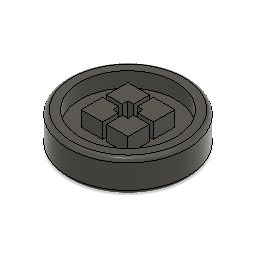
DC801-BM-Joy-Hats-symbols v13 (Autodesk Fusion 360 design; units mm, degrees)
Autodesk Fusion 360 part; units mm, degrees
note: some values were not read from the file. Chosen so that the rebuilt part matches the saved one: which bodies a step acts on; which face or edge a step refers to. Set by a fixed rule: which sketch regions a step uses.
sketch "Sketch1" plane through (0, 0, 0) normal (0, 1, 0) x (1, 0, 0)
  line L0 (0.95, 0.95) -> (-0.95, 0.95)
  line L1 (-0.95, 0.95) -> (-0.95, -0.95)
  line L2 (-0.95, -0.95) -> (0.95, -0.95)
  line L3 (0.95, -0.95) -> (0.95, 0.95)
  line L4 (0.95, 0.95) -> (-0.95, -0.95) construction
  line L5 (-0.95, 0.95) -> (0.95, -0.95) construction
  circle A0 centre (0, 0) radius 7.5
  line L6 (0.25, -2.95) -> (-0.25, -2.95)
  line L7 (-0.25, -2.95) -> (-0.25, 2.95)
  line L8 (-0.25, 2.95) -> (0.25, 2.95)
  line L9 (0.25, 2.95) -> (0.25, -2.95)
  line L10 (0.25, -2.95) -> (-0.25, 2.95) construction
  line L11 (-0.25, -2.95) -> (0.25, 2.95) construction
  line L12 (2.95, 2.95) -> (-2.95, 2.95)
  line L13 (-2.95, 2.95) -> (-2.95, -2.95)
  line L14 (-2.95, -2.95) -> (2.95, -2.95)
  line L15 (2.95, -2.95) -> (2.95, 2.95)
  circle A1 centre (0, 0) radius 6
  line L16 (2.95, 0.25) -> (-2.95, 0.25)
  line L17 (-2.95, 0.25) -> (-2.95, -0.25)
  line L18 (-2.95, -0.25) -> (2.95, -0.25)
  line L19 (2.95, -0.25) -> (2.95, 0.25)
  line L20 (2.95, 0.25) -> (-2.95, -0.25) construction
  line L21 (-2.95, 0.25) -> (2.95, -0.25) construction
  dimension "d1" = 1.9
  dimension "d2" = 1.9
  dimension "d3" = 15
  dimension "d35" = 0.5
  dimension "d63" = 2
  dimension "d68" = 2
  dimension "d71" = 0.5
  dimension "d94" = 5.9
  dimension "d96" = 5.9
  constraint horizontal L0
  constraint perpendicular L0 L1
  constraint parallel L0 L2
  constraint parallel L1 L3
  constraint coincident L4 A0.centre
  constraint coincident L5 A0.centre
  constraint coincident A0.centre A1.centre
  constraint horizontal L6
  constraint perpendicular L6 L7
  constraint parallel L6 L8
  constraint parallel L7 L9
  constraint coincident L10 A0.centre
  constraint coincident L11 A0.centre
  constraint horizontal L16
  constraint perpendicular L16 L17
  constraint parallel L16 L18
  constraint parallel L17 L19
  constraint coincident L20 A0.centre
  constraint coincident L21 A0.centre
  measures "d1" distance of L1.end L2.end
  measures "d2" distance of L0.end L1.end
  measures "d3" diameter of A0
  measures "d35" distance of L7.end L8.end
  measures "d63" distance of L2 L6
  measures "d71" distance of L16.end L17.end
  measures "d94" distance of L16.start L16.end
  measures "d96" distance of L6.start L8.end
extrude "Extrude1" add sketch "Sketch1" along normal blind 3 contours L0 L3 L9 L12 L15 L16 | L0 L1 L7 L12 L13 L16 | L2 L3 L9 L14 L15 L18 | L1 L2 L7 L13 L14 L18 | A0 makes body 1 at (2.95, 1, -1.15) makes body 2 at (2.95, 1, 2.05) makes body 3 at (-1.15, 1, -2.95) makes body 4 at (7.4907, 2, 0.3738) makes body 5 at (-2.95, 1, 1.15)
extrude "Extrude12" add sketch "Sketch1" against normal blind 1 contours L0 L3 L9 L16 | L0 L3 L9 L12 L15 L16 | L0 L7 L9 L16 | L0 L7 L8 L9 L12 | L3 L15 L16 L18 L19 | L3 L9 L16 L18 | L0 L1 L7 L16 | L0 L1 L7 L12 L13 L16 | L7 L9 L16 L18 | L2 L3 L9 L14 L15 L18 | L2 L3 L9 L18 | L1 L7 L16 L18 | L2 L7 L9 L18 | L1 L13 L16 L17 L18 | L1 L2 L7 L18 | L2 L6 L7 L9 L14 | L1 L2 L7 L13 L14 L18 | A0 | A1 bodies 1 2 3 4 5
sketch "Sketch17" plane through (0, 0, 0) normal (0, 1, 0) x (-1, 0, 0)
  line L0 (-2.95, -2.95) -> (-2.95, -0.25)
  line L1 (-2.95, -0.25) -> (-0.95, -0.25)
  line L2 (-0.95, -0.25) -> (-0.95, -0.95)
  line L3 (-0.95, -0.95) -> (-0.25, -0.95)
  line L4 (-0.25, -0.95) -> (-0.25, -2.95)
  line L5 (-0.25, -2.95) -> (-2.95, -2.95)
  line L6 (2.95, -2.95) -> (0.25, -2.95)
  line L7 (0.25, -2.95) -> (0.25, -0.95)
  line L8 (0.25, -0.95) -> (0.95, -0.95)
  line L9 (0.95, -0.95) -> (0.95, -0.25)
  line L10 (0.95, -0.25) -> (2.95, -0.25)
  line L11 (2.95, -0.25) -> (2.95, -2.95)
  line L12 (2.95, 2.95) -> (2.95, 0.25)
  line L13 (2.95, 0.25) -> (0.95, 0.25)
  line L14 (0.95, 0.25) -> (0.95, 0.95)
  line L15 (0.95, 0.95) -> (0.25, 0.95)
  line L16 (0.25, 0.95) -> (0.25, 2.95)
  line L17 (0.25, 2.95) -> (2.95, 2.95)
  line L18 (-2.95, 2.95) -> (-0.25, 2.95)
  line L19 (-0.25, 2.95) -> (-0.25, 0.95)
  line L20 (-0.25, 0.95) -> (-0.95, 0.95)
  line L21 (-0.95, 0.95) -> (-0.95, 0.25)
  line L22 (-0.95, 0.25) -> (-2.95, 0.25)
  line L23 (-2.95, 0.25) -> (-2.95, 2.95)
  line L24 (-2.95, -2.95) -> (2.95, -2.95)
  line L25 (2.95, -2.95) -> (2.95, 2.95)
  line L26 (2.95, 2.95) -> (-2.95, 2.95)
  line L27 (-2.95, 2.95) -> (-2.95, -2.95)
  line L28 (-2.95, -2.95) -> (2.95, 2.95) construction
  line L29 (2.95, -2.95) -> (-2.95, 2.95) construction
  circle A0 centre (0, 0) radius 6
  dimension "d103" = 5.9
  dimension "d104" = 5.9
  constraint horizontal L24
  constraint perpendicular L24 L25
  constraint parallel L24 L26
  constraint parallel L25 L27
  constraint coincident L28 A0.centre
  constraint coincident L29 A0.centre
  measures "d103" distance of L12.start L18.start
  measures "d104" distance of L6.start L12.start
extrude "Extrude18" add sketch "Sketch17" along normal blind 1.1 contours L1 L2 L3 L4 L7 L8 L9 L10 L13 L14 L15 L16 L19 L20 L21 L22 L24 L25 L26 L27 bodies 1
sketch "Sketch18" plane through (0, -1, 0) normal (0, -1, 0) x (1, 0, 0)
  line L0 (6.5, 1.5) -> (-6.5, 1.5)
  line L1 (-6.5, 1.5) -> (-6.5, -1.5)
  line L2 (-6.5, -1.5) -> (6.5, -1.5)
  line L3 (6.5, -1.5) -> (6.5, 1.5)
  line L4 (6.5, 1.5) -> (-6.5, -1.5) construction
  line L5 (-6.5, 1.5) -> (6.5, -1.5) construction
  line L6 (-3.5, 1.5) -> (-3.5, -1.5)
  line L7 (-3.5, 0) -> (-6.5, 0) construction
  line L8 (-3.8606, 0.9565) -> (-6.1403, -0.9573) construction
  line L9 (-6.1151, 1.0426) -> (-4.1467, -0.7978) construction
  circle A0 centre (5, 0) radius 1.5
  line L10 (-0.012, 6.5) -> (-1.7598, 3.5092)
  line L11 (-1.7598, 3.5092) -> (1.7042, 3.4909)
  line L12 (1.7042, 3.4909) -> (-0.012, 6.5)
  circle A1 centre (5, 0) radius 1.1
  line L13 (-4, 1) -> (-6, 1)
  line L14 (-6, 1) -> (-6, -1)
  line L15 (-6, -1) -> (-4, -1)
  line L16 (-4, -1) -> (-4, 1)
  line L17 (-4, 1) -> (-6, -1) construction
  line L18 (-6, 1) -> (-4, -1) construction
  line L19 (-0.0147, 6) -> (-1.3255, 3.7569)
  line L20 (-1.3255, 3.7569) -> (1.2725, 3.7432)
  line L21 (1.2725, 3.7432) -> (-0.0147, 6)
  line L22 (1, -4) -> (-1, -4) construction
  line L23 (-1, -4) -> (-1, -6) construction
  line L24 (-1, -6) -> (1, -6) construction
  line L25 (1, -6) -> (1, -4) construction
  line L26 (1, -4) -> (-1, -6) construction
  line L27 (-1, -4) -> (1, -6) construction
  line L28 (-1, -5.6818) -> (0.6818, -4)
  line L29 (-0.6818, -6) -> (1, -4.3182)
  line L30 (-0.6818, -4) -> (1, -5.6818)
  line L31 (-1, -4.3182) -> (0.6818, -6)
  line L32 (1.5, -3.5) -> (-1.5, -3.5)
  line L33 (-1.5, -3.5) -> (-1.5, -6.5)
  line L34 (-1.5, -6.5) -> (1.5, -6.5)
  line L35 (1.5, -6.5) -> (1.5, -3.5)
  line L36 (1.5, -3.5) -> (-1.5, -6.5) construction
  line L37 (-1.5, -3.5) -> (1.5, -6.5) construction
  line L38 (0.6818, -4) -> (1.1818, -3.5)
  line L39 (1, -4.3182) -> (1.5, -3.8182)
  line L40 (-0.6818, -4) -> (-1.1818, -3.5)
  line L41 (-1, -4.3182) -> (-1.5, -3.8182)
  line L42 (-1, -5.6818) -> (-1.5, -6.1818)
  line L43 (-0.6818, -6) -> (-1.1818, -6.5)
  line L44 (0.6818, -6) -> (1.1818, -6.5)
  line L45 (1, -5.6818) -> (1.5, -6.1818)
  circle A2 centre (0, 0) radius 7.5
  point P0 (-5, 0)
  point P1 (-0.0226, 4.5)
  point P2 (-5, 0)
  point P3 (-0.0226, 4.5)
  point P4 (0, -5)
  point P5 (0, -5)
  dimension "d110" = 3
  dimension "d111" = 3
  dimension "d112" = 2
  dimension "d113" = 2
  dimension "d114" = 1.5
  dimension "d115" = 1.5
  dimension "d122" = 0.4
  dimension "d123" = 0.5
  dimension "d124" = 0.5
  dimension "d125" = 0.25
  dimension "d126" = 13
  dimension "d129" = 3
  dimension "d131" = 6.5
  dimension "d136" = 3
  dimension "d137" = 2
  dimension "d138" = 2
  dimension "d140" = 0.225
  dimension "d141" = 0.225
  dimension "d142" = 0.225
  dimension "d143" = 0.225
  dimension "d148" = 3
  dimension "d149" = 3
  dimension "d150" = 6.5
  constraint horizontal L0
  constraint perpendicular L0 L1
  constraint parallel L0 L2
  constraint parallel L1 L3
  constraint coincident L4 A2.centre
  constraint coincident L5 A2.centre
  constraint coincident A2.centre origin
  constraint coincident L0 L6.start
  constraint coincident L2 L6.end
  constraint perpendicular L2 L6
  constraint midpoint L6 L7.start
  constraint midpoint L1 L7.end
  constraint coincident L8 P2
  constraint coincident L9 P2
  constraint midpoint L7 P2
  constraint tangent L0 A0
  constraint concentric A0 A1
  constraint horizontal L13
  constraint perpendicular L13 L14
  constraint parallel L13 L15
  constraint parallel L14 L16
  constraint coincident L17 P2
  constraint coincident L18 P2
  constraint coincident P2 P0
  constraint coincident P3 P1
  constraint horizontal L22
  constraint perpendicular L22 L23
  constraint parallel L22 L24
  constraint parallel L23 L25
  constraint coincident L26 P5
  constraint coincident L27 P5
  constraint coincident L23 L28.start
  constraint coincident L22 L28.end
  constraint perpendicular L27 L28
  constraint coincident L24 L29.start
  constraint coincident L25 L29.end
  constraint parallel L28 L29
  constraint coincident L22 L30.start
  constraint coincident L25 L30.end
  constraint perpendicular L29 L30
  constraint coincident L23 L31.start
  constraint coincident L24 L31.end
  constraint perpendicular L29 L31
  constraint horizontal L32
  constraint perpendicular L32 L33
  constraint parallel L32 L34
  constraint parallel L33 L35
  constraint coincident L36 P5
  constraint coincident L37 P5
  constraint coincident P5 P4
  constraint coincident L32 L38.end
  constraint parallel L28 L38
  constraint coincident L35 L39.end
  constraint parallel L29 L39
  constraint coincident L32 L40.end
  constraint perpendicular L39 L40
  constraint coincident L33 L41.end
  constraint parallel L31 L41
  constraint perpendicular L41 L42
  constraint coincident L34 L43.end
  constraint parallel L29 L43
  constraint coincident L34 L44.end
  constraint parallel L31 L44
  constraint coincident L35 L45.end
  constraint parallel L31 L45
  measures "d110" distance of L0.end L1.end
  measures "d111" distance of L1 L6
  measures "d112" distance of L8.end L9.end
  measures "d113" distance of L9.start L8.end
  measures "d114" distance of L7.end P2
  measures "d115" distance of L3 A0.centre
  measures "d122" distance of A0 A1
  measures "d123" distance of L0 L13
  measures "d124" distance of L6 L16
  measures "d125" distance of L12 L21
  measures "d126" distance of L0.start L0.end
  measures "d129" diameter of A0
  measures "d131" vertical distance of A2.centre L10.start
  measures "d136" distance of L10.start L11
  measures "d137" distance of L23.end L24.end
  measures "d138" distance of L22.end L23.end
  measures "d140" distance of L26 L28
  measures "d141" distance of L26 L29
  measures "d142" distance of L27 L30
  measures "d143" distance of L27 L31
  measures "d148" distance of L33.end L34.end
  measures "d149" distance of L32.end L33.end
  measures "d150" distance of A2.centre L34
extrude "Extrude19" cut sketch "Sketch18" against normal blind 0.8 contours L0 L1 L2 L6 | A0 | L10 L11 L12 | A1 | L13 L14 L15 L16 | L19 L20 L21 | L28 L29 L31 L33 L34 L42 L43 | L28 L30 L31 L32 L33 L40 L41 | L28 L29 L30 L31 | L28 L29 L30 L32 L35 L38 L39 | L29 L30 L31 L34 L35 L44 L45 bodies 1
extrude "Extrude20" add sketch "Sketch18" against normal blind 0.2 separate body contours L0 L1 L2 L6 | A0 | L10 L11 L12 | A1 | L13 L14 L15 L16 | L19 L20 L21 | L28 L29 L31 L33 L34 L42 L43 | L28 L30 L31 L32 L33 L40 L41 | L28 L29 L30 L31 | L28 L29 L30 L32 L35 L38 L39 | L29 L30 L31 L34 L35 L44 L45 makes body 6 at (-0.0226, -1, 4.5) makes body 7 at (0.8939, -1, -4) makes body 8 at (-4.5, -1, -0.5) makes body 9 at (5.2951, -1, 0.3621)
fillet "Fillet6" radius 0.5 1 edges at (-6.9925, -1, -2.7121) on bodies 1
fillet "Fillet7" radius 0.5 1 edges at (-6.9925, 3, 2.7121) on bodies 1
combine "Combine1" operation add target body 8 tool bodies 9 6 7 makes body 10 at (-0.0226, -1, 4.5) makes body 11 at (5.2951, -1, 0.3621) makes body 12 at (0.8939, -1, -4)
extrude "Extrude21" add 1 faces at (3.9667, 0, 0) along direction (0, 1, 0) blind 1.1 on bodies 1 bodies 1
hidden bodies 8 10 11 12
